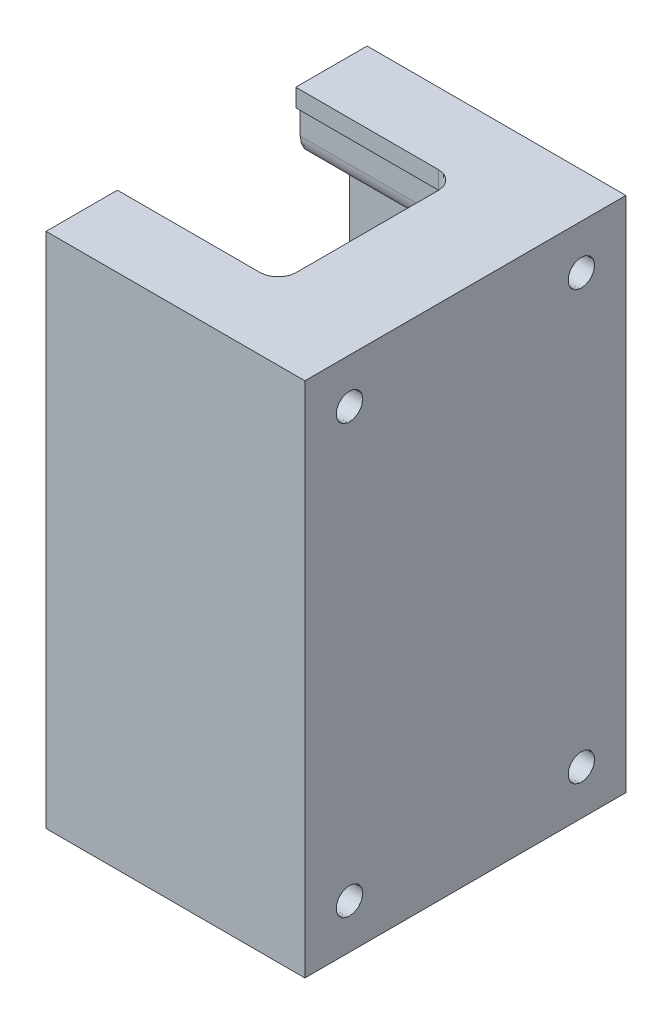
# Autodesk Inventor part: enclosure
Saved by Autodesk Inventor 2021 (Build 250183000, 183)
## iProperties
Created: 2021-08-23
Part Number: enclosure
Material: Generic
Document SubType Name: Modeling
Designer: techv
Density: 1 g/cm^3
Appearance: Default
Author: techv
Autodesk Inventor part; units mm, degrees
ref_plane "YZ Plane" through (0, 0, 0) normal (1, 0, 0) x (0, 1, 0)
ref_plane "XZ Plane" through (0, 0, 0) normal (0, 1, 0) x (-1, 0, 0)
ref_plane "XY Plane" through (0, 0, 0) normal (0, 0, 1) x (1, 0, 0)
ref_plane "Work Plane1" through (13.6834, 18.9252, 14.6894) normal (1, 0, 0) x (0, 1, 0)
sketch "Sketch1" plane through (13.6834, 18.9252, 14.6894) normal (1, 0, 0) x (0, 1, 0)
  circle A0 centre (3, 27.9806) radius 1.5 projected
  circle A1 centre (3, 1.9806) radius 1.5 projected
  circle A2 centre (-45, 1.9806) radius 1.5 projected
  circle A3 centre (-45, 27.9806) radius 1.5 projected
  line L0 (-50, 32.9806) -> (8, 32.9806) projected
  line L1 (8, 32.9806) -> (8, 24.9805) projected
  line L2 (8, -3.0194) -> (8, 4.9808) projected
  line L3 (-50, -3.0194) -> (8, -3.0194) projected
  line L4 (-50, 0) -> (-50, 32.9806) projected
  line L5 (-50, -0.0388) -> (-50, -3.0194) projected
  line L6 (100, 24.9806) -> (0, 24.9806) projected
  line L7 (0, 22.9806) -> (0, 24.9806) projected
  line L8 (0, 22.9806) -> (0, 6.9806) projected
  line L9 (0, 4.9806) -> (0, 6.9806) projected
  line L10 (0, 4.9806) -> (100, 4.9806) projected
  line L11 (6, 24.9806) -> (6, 25.4806)
  line L12 (0.5, 30.9806) -> (-42.5, 30.9806)
  line L13 (-48, 25.4806) -> (-48, 4.4806)
  line L14 (-42.5, -1.0194) -> (0.5, -1.0194)
  line L15 (6, 4.4806) -> (6, 4.9806)
  arc A4 (0.5, 27.9806) -> (3, 25.4806) centre (3, 27.9806) ccw
  arc A5 (3, 4.4806) -> (0.5, 1.9806) centre (3, 1.9806) ccw
  arc A6 (-42.5, 1.9806) -> (-45, 4.4806) centre (-45, 1.9806) ccw
  arc A7 (-45, 25.4806) -> (-42.5, 27.9806) centre (-45, 27.9806) ccw
  line L16 (-45, 25.4806) -> (-48, 25.4806)
  line L17 (-42.5, 27.9806) -> (-42.5, 30.9806)
  line L18 (-45, 4.4806) -> (-48, 4.4806)
  line L19 (-42.5, 1.9806) -> (-42.5, -1.0194)
  line L20 (0.5, 1.9806) -> (0.5, -1.0194)
  line L21 (3, 4.4806) -> (6, 4.4806)
  line L22 (0.5, 27.9806) -> (0.5, 30.9806)
  line L23 (3, 25.4806) -> (6, 25.4806)
  circle A8 centre (-45, 1.9806) radius 1.5
  circle A9 centre (-45, 27.9806) radius 1.5
  circle A10 centre (3, 27.9806) radius 1.5
  circle A11 centre (3, 1.9806) radius 1.5
  line L24 (8, 4.9808) -> (8, -3.0194)
  line L25 (-50, -3.0194) -> (8, -3.0194)
  line L26 (-50, -3.0194) -> (-50, 32.9806)
  line L27 (8, 32.9806) -> (-50, 32.9806)
  line L28 (8, 24.9805) -> (8, 32.9806)
  line L29 (8, 24.9805) -> (0, 24.9806)
  line L30 (0, 4.9806) -> (0, 24.9806)
  line L31 (0, 4.9806) -> (8, 4.9808)
  point P0 (-18.9252, -14.6894)
  point P1 (8, 24.9806)
  point P2 (8, 4.9806)
  dimension "d0" = 2
  dimension "d1" = 2
  dimension "d2" = 2
  dimension "d3" = 2
  dimension "d4" = 2
  dimension "d5" = 5
  dimension "d6" = 5
  dimension "d7" = 5
  dimension "d8" = 5
  constraints: 42 end point, 11 perpendicular, 9 point on line, 8 centre point, 8 coincident, 8 point on circle, 5 tangent, 4 concentric, 2 vertical, 1 parallel
  measures "d0" distance between parallel lines of L0 L12
  measures "d1" distance between parallel lines of L11 L1
  measures "d2" distance between parallel lines of L15 L2
  measures "d3" distance between parallel lines of L3 L14
  measures "d4" distance between parallel lines of L4 L13
  measures "d5" diameter of A4
  measures "d6" diameter of A5
  measures "d7" diameter of A6
  measures "d8" diameter of A7
extrude "Extrusion1" add sketch "Sketch1" along normal blind 26.024 contours L0 L1 L6 L11 L23 A4 L22 L12 L17 A7 L16 L13 L18 A6 L19 L14 L20 A5 L21 L15 L10 L2 L3 L5 L26 L4
sketch "Sketch2" plane through (13.6834, -31.0748, 11.67) normal (0, 0, -1) x (-1, 0, 0)
  line L0 (0, 0) -> (-26.024, 0) projected
  line L1 (-26.024, 0) -> (-29.024, 0)
  line L2 (-29.024, 0) -> (-29.024, 58)
  line L3 (-29.024, 58) -> (-25.5921, 58)
  line L4 (-26.024, 0) -> (-26.024, 58) projected
  line L5 (-26.024, 0) -> (-26.024, 58)
  point P0 (13.6834, 31.0748)
  dimension "d11" = 3
  dimension "d12" = 58
  constraints: 8 end point, 2 perpendicular, 1 horizontal, 1 vertical
  measures "d11" distance of L0.end L1.end
  measures "d12" distance of L1.end L2.end
extrude "Extrusion2" add sketch "Sketch2" against normal up to surface (36 mm away)
sketch "Sketch3" plane through (42.7074, -31.0748, 11.67) normal (1, 0, 0) x (0, 0, -1)
  point P0 (11.67, 31.0748)
sketch "Sketch4" plane through (42.7074, -31.0748, 11.67) normal (1, 0, 0) x (0, 0, -1)
  circle A0 centre (-31, 53) radius 1.5 projected
  circle A1 centre (-5, 53) radius 1.5 projected
  circle A2 centre (-5, 5) radius 1.5 projected
  circle A3 centre (-31, 5) radius 1.5 projected
  point P0 (11.67, 31.0748)
extrude "Extrusion3" cut sketch "Sketch4" against normal through all
sketch "Sketch5" plane through (13.6834, 26.9252, 47.67) normal (0, 1, 0) x (1, 0, 0)
  line L0 (18.024, 10) -> (18.024, 26) projected
  arc A0 (18.024, 26) -> (16.024, 28) centre (16.024, 26) ccw projected
  arc A1 (16.024, 8) -> (18.024, 10) centre (16.024, 10) ccw projected
  line L1 (0.024, 8) -> (16.024, 8) projected
  line L2 (16.024, 28) -> (0.024, 28) projected
  line L3 (0, 8) -> (0, 0) projected
  line L4 (0, 0) -> (29.024, 0) projected
  line L5 (29.024, 36) -> (29.024, 0) projected
  line L6 (0, 36) -> (29.024, 36) projected
  line L7 (0, 36) -> (0, 28) projected
  line L8 (0, 28) -> (26.024, 28) projected
  line L9 (26.024, 28) -> (26.024, 8) projected
  line L10 (0, 8) -> (26.024, 8) projected
  point P0 (-13.6834, 47.67)
  point P1 (16.024, 8)
extrude "Extrusion4" add sketch "Sketch5" against normal blind 2 contours L0 A0 L8 L9 L10 A1
body "Solid1"
